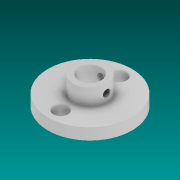
# Autodesk Inventor part: asbevestiging
Saved by Autodesk Inventor 2020.2 (Build 242310000, 310)
## iProperties
Created: 2020-05-20
Part Number: asbevestiging
Material: Aluminum 6061
Document SubType Name: Modeling
Designer: Svend
Density: 2.7 g/cm^3
Appearance: Aluminum - Polished
Author: Svend
Autodesk Inventor part; units mm, degrees
ref_plane "YZ Plane" through (0, 0, 0) normal (1, 0, 0) x (0, 1, 0)
ref_plane "XZ Plane" through (0, 0, 0) normal (0, 1, 0) x (-1, 0, 0)
ref_plane "XY Plane" through (0, 0, 0) normal (0, 0, 1) x (1, 0, 0)
sketch "Sketch1" plane through (0, 0, 0) normal (0, 0, 1) x (1, 0, 0)
  line L0 (0, 10) -> (6, 10)
  line L1 (6, 10) -> (6, 4)
  line L2 (6, 4) -> (15, 4)
  line L3 (15, 4) -> (15, 0)
  line L4 (15, 0) -> (0, 0)
  line L5 (0, 0) -> (0, 10)
  dimension "d0" = 4
  dimension "d1" = 10
  dimension "d2" = 15
  dimension "d3" = 6
  constraints: 12 end point, 5 perpendicular, 1 horizontal
  measures "d0" distance of L2.end L3.end
  measures "d1" distance between parallel lines of L0 L4
  measures "d2" distance between parallel lines of L3 L5
  measures "d3" distance between parallel lines of L5 L1
revolve "Revolution1" add sketch "Sketch1" angle 360 about axis through (0, 0, 0) along (0, 1, 0)
sketch "Sketch2" plane through (0, 10, 0) normal (0, 1, 0) x (1, 0, 0)
  circle A0 centre (0, 0) radius 6 projected
  line L0 (0, 6) -> (0, 15)
  circle A1 centre (0, 0) radius 15 projected
  circle A2 centre (0, 0) radius 6 projected
  circle A3 centre (0, 0) radius 15 projected
  line L1 (0, -6) -> (0, -15)
  point P0 (0, 10.5)
  point P1 (0, -10.5)
  point P2 (0, -10.5)
  point P3 (0, 10.5)
  constraints: 5 coincident, 4 end point, 4 vertical alignment, 2 midpoint, 2 point on line, 2 vertical, 4 other
hole "Hole1" at (0, 10, 0) direction (0, -1, 0) diameter 8 end through all
hole "Hole2" at (0, 10, -10.5) at (0, 10, 10.5) direction (0, -1, 0) diameter 5.2 end through all
sketch "Sketch3" plane through (0, 0, 0) normal (1, 0, 0) x (0, 1, 0)
  line L0 (10, 6) -> (10, -6) projected
  line L1 (4, 6) -> (4, -6) projected
  line L2 (4, 15) -> (4, -15) projected
  line L3 (0, 15) -> (0, -15) projected
  line L4 (10, 0) -> (4, 0)
  line L5 (4, 6) -> (4, -6) projected
  point P0 (0, 0)
  point P1 (7, 0)
  point P2 (7, 0)
  constraints: 3 midpoint, 2 coincident, 2 end point
hole "Hole3" at (0, 7, 0) direction (1, 0, 0) diameter 2.459 end through all thread size "M3x0.5" class "6H" standard "ISO Metric profile"
sketch "Sketch4" plane through (0, 0, 0) normal (0, 0, 1) x (1, 0, 0)
  line L0 (-15, 4) -> (15, 4) projected
  line L1 (-15, 0) -> (15, 0) projected
  line L2 (-4, 10) -> (4, 10) projected
  line L3 (0, 10) -> (0, 4)
  line L4 (-6, 4) -> (6, 4) projected
  point P0 (0, 0)
  point P1 (0, 7)
  constraints: 3 midpoint, 2 end point
hole "Hole4" at (0, 7, 0) direction (0, 0, -1) diameter 2.459 end through all thread size "M3x0.5" class "6H" standard "ISO Metric profile"
body "Solid1"
